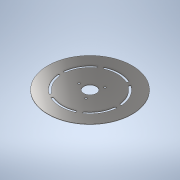
# Autodesk Inventor part: Tarcza_Okładzina
Saved by Autodesk Inventor 2022 (Build 260153000, 153)
## iProperties
Created: 2021-06-19
Part Number: Tarcza_Okładzina
Material: Stal, węglowa
Document SubType Name: Modeling
Designer: Matik
Density: 7.85 g/cm^3
Appearance: Częściowo polerowany
Author: Matik
Autodesk Inventor part; units mm, degrees
ref_plane "YZ Plane" through (0, 0, 0) normal (1, 0, 0) x (0, 1, 0)
ref_plane "XZ Plane" through (0, 0, 0) normal (0, 1, 0) x (-1, 0, 0)
ref_plane "XY Plane" through (0, 0, 0) normal (0, 0, 1) x (1, 0, 0)
sketch "Szkic1" plane through (0, 0, 0) normal (0, 1, 0) x (-1, 0, 0)
  circle A0 centre (0, 0) radius 15
  circle A1 centre (0, 0) radius 40
  circle A2 centre (0, 0) radius 100
  circle A3 centre (0, 0) radius 70
  circle A4 centre (0, 0) radius 65
  line L0 (70, 0) -> (65, 0)
  arc A5 (64.5545, 7.5974) -> (69.7435, 5.9875) centre (67.5065, 7.9448) ccw
  arc A6 (69.7385, -6.0444) -> (64.5482, -7.6502) centre (67.5, -8) ccw
  arc A7 (40.1039, 57.3731) -> (38.8994, 52.0753) centre (40.6782, 54.4567) ccw
  arc A8 (25.6977, 59.7045) -> (29.6864, 63.3933) centre (26.8728, 62.4348) ccw
  arc A9 (-29.6346, 63.4176) -> (-25.6489, 59.7255) centre (-26.8218, 62.4567) ccw
  arc A10 (-38.8568, 52.1071) -> (-40.057, 57.4059) centre (-40.6337, 54.4899) ccw
  arc A11 (-69.7385, 6.0444) -> (-64.5482, 7.6502) centre (-67.5, 8) ccw
  arc A12 (-64.5545, -7.5974) -> (-69.7435, -5.9875) centre (-67.5065, -7.9448) ccw
  arc A13 (-40.1039, -57.3731) -> (-38.8994, -52.0753) centre (-40.6782, -54.4567) ccw
  arc A14 (-25.6977, -59.7045) -> (-29.6864, -63.3933) centre (-26.8728, -62.4348) ccw
  arc A15 (29.6346, -63.4176) -> (25.6489, -59.7255) centre (26.8218, -62.4567) ccw
  arc A16 (38.8568, -52.1071) -> (40.057, -57.4059) centre (40.6337, -54.4899) ccw
  point P0 (-29.6346, 63.4176)
  point P1 (29.6864, 63.3933)
  point P2 (-38.8568, 52.1071)
  point P3 (-69.7385, 6.0444)
  point P4 (-40.1039, -57.3731)
  point P5 (-69.7435, -5.9875)
  point P6 (29.6346, -63.4176)
  point P7 (-29.6864, -63.3933)
  point P8 (38.8568, -52.1071)
  point P9 (40.057, -57.4059)
  point P10 (38.8994, 52.0753)
  point P11 (40.1039, 57.3731)
  dimension "d0" = 30
  dimension "d20" = 200
  dimension "d21" = 140
  dimension "d22" = 130
  dimension "d25" = 10
  dimension "d28" = 360
  constraints: 30 point on circle, 17 centre point, 4 coincident, 2 end point, 2 tangent, 1 horizontal, 49 other
  measures "d0" diameter of A0
  measures "d20" diameter of A2
  measures "d21" diameter of A3
  measures "d22" diameter of A4
extrude "Wyciągnięcie proste1" add sketch "Szkic1" along normal blind 1 contours A1 | A2 | L0 A4 A5 A3 | A3 A6 A4 L0 | A4 | A7 A4 A8 A3 | A3 A15 A4 A16 | A9 A4 A10 A3 | A3 A13 A4 A14 | A11 A4 A12 A3
sketch "Szkic3" plane through (0, 1, 0) normal (0, 1, 0) x (1, 0, 0)
  circle A0 centre (0, 0) radius 22.5
  circle A1 centre (-26, 0) radius 2.5
  circle A2 centre (13, -22.5167) radius 2.5
  circle A3 centre (13, 22.5167) radius 2.5
  dimension "d42" = 45
  dimension "d46" = 5
  dimension "d50" = 360
  dimension "d54" = 26
  constraints: 4 centre point, 1 coincident, 7 other
  measures "d42" diameter of A0
  measures "d46" diameter of A1
  measures "d54" distance of A0.centre A1.centre
extrude "Wyciągnięcie proste3" cut sketch "Szkic3" against normal blind 10 contours A1 | A2 | A3
sketch "Szkic4" plane through (0, 1, 0) normal (0, 1, 0) x (1, 0, 0)
  point P0 (0, 0)
